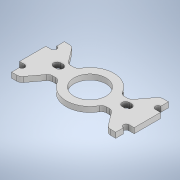
# Autodesk Inventor part: Ankle_middle_frame
Saved by Autodesk Inventor 2020.4 (Build 244396000, 396)
## iProperties
Created: 2021-10-01
Part Number: Ankle_middle_frame
Material: アルミニウム 2014-T4
Document SubType Name: Modeling
Designer: Masato Kubotera
Density: 2.8 g/cm^3
Appearance: 滑らか - 淡い灰色
Description: A2017 T2
Author: Masato Kubotera
Autodesk Inventor part; units mm, degrees
ref_plane "YZ Plane" through (0, 0, 0) normal (1, 0, 0) x (0, 1, 0)
ref_plane "XZ Plane" through (0, 0, 0) normal (0, 1, 0) x (-1, 0, 0)
ref_plane "XY Plane" through (0, 0, 0) normal (0, 0, 1) x (1, 0, 0)
sketch "スケッチ1" plane through (0, 0, 0) normal (0, 0, 1) x (1, 0, 0)
  line L0 (-19.75, 10) -> (19.75, 10) construction
  line L1 (19.75, 10) -> (19.75, -10) construction
  line L2 (19.75, -10) -> (-19.75, -10) construction
  line L3 (-19.75, -10) -> (-19.75, 10) construction
  line L4 (-19.75, 10) -> (19.75, -10) construction
  line L5 (19.75, 10) -> (-19.75, -10) construction
  line L6 (-19.75, 5) -> (-21.75, 5)
  line L7 (-21.75, 5) -> (-21.75, -5)
  line L8 (-19.75, 0) -> (19.75, 0) construction
  line L9 (0, 10) -> (0, -10) construction
  arc A0 (-19.75, 5) -> (-19.75, 7.1) centre (-19.75, 6.05) ccw
  line L10 (-16.75, 10) -> (-11.75, 3.4)
  line L11 (-19.75, -5) -> (-21.75, -5)
  arc A1 (-19.75, -7.1) -> (-19.75, -5) centre (-19.75, -6.05) ccw
  line L12 (-16.75, -10) -> (-11.75, -3.4)
  line L13 (-19.75, 7.1) -> (-19.75, 10)
  line L14 (-16.75, 10) -> (-19.75, 10)
  line L15 (-16.75, -10) -> (-19.75, -10)
  line L16 (-19.75, -7.1) -> (-19.75, -10)
  line L17 (19.75, 5) -> (21.75, 5)
  line L18 (21.75, 5) -> (21.75, -5)
  arc A2 (19.75, 7.1) -> (19.75, 5) centre (19.75, 6.05) ccw
  line L19 (16.75, 10) -> (11.75, 3.4)
  line L20 (19.75, -5) -> (21.75, -5)
  arc A3 (19.75, -5) -> (19.75, -7.1) centre (19.75, -6.05) ccw
  line L21 (16.75, -10) -> (11.75, -3.4)
  line L22 (19.75, 7.1) -> (19.75, 10)
  line L23 (16.75, 10) -> (19.75, 10)
  line L24 (16.75, -10) -> (19.75, -10)
  line L25 (19.75, -7.1) -> (19.75, -10)
  arc A4 (8.387, 3.4) -> (-8.387, 3.4) centre (0, 0) ccw
  arc A5 (-8.387, -3.4) -> (8.387, -3.4) centre (0, 0) ccw
  line L26 (-11.75, 3.4) -> (-8.387, 3.4)
  line L27 (-8.387, -3.4) -> (-11.75, -3.4)
  line L28 (8.387, -3.4) -> (11.75, -3.4)
  line L29 (11.75, 3.4) -> (8.387, 3.4)
  circle A6 centre (0, 0) radius 6 construction
  circle A7 centre (0, 0) radius 6.05
  arc A8 (-13.5, 2.35) -> (-13.5, -0.35) centre (-13.5, 1) ccw
  line L30 (-13.5, 1) -> (13.5, 1) construction
  line L31 (-13.5, 2.35) -> (-12.5, 2.35)
  line L32 (-12.5, -0.35) -> (-13.5, -0.35)
  arc A9 (-12.5, -0.35) -> (-12.5, 2.35) centre (-12.5, 1) ccw
  circle A10 centre (-13.5, 1) radius 2.4 construction
  arc A11 (13.5, -0.35) -> (13.5, 2.35) centre (13.5, 1) ccw
  arc A12 (12.5, 2.35) -> (12.5, -0.35) centre (12.5, 1) ccw
  line L33 (12.5, 2.35) -> (13.5, 2.35)
  line L34 (12.5, -0.35) -> (13.5, -0.35)
  point P0 (0, 0)
  point P1 (0, 1)
  dimension "d0" = 39.5
  dimension "d4" = 2
  dimension "d5" = 10
  dimension "d6" = 1.05
  dimension "d7" = 3
  dimension "d9" = 5
  dimension "d11" = 8
  dimension "d26" = 12
  dimension "d27" = 0.05
  dimension "d28" = 12.1
  dimension "d30" = 27
  dimension "d32" = 1
  dimension "d33" = 1.35
  dimension "d34" = 1
  dimension "d35" = 4.8
  dimension "d36" = 3
  constraints: 70 end point, 26 symmetric about line, 20 point on circle, 13 centre point, 11 midpoint, 6 parallel, 6 point on line, 5 horizontal, 5 tangent, 3 coincident, 3 perpendicular, 2 collinear, 6 other
  measures "d0" distance of L1.end L2.end
  measures "d4" distance of L6.start L6.end
  measures "d5" distance of L6.end L7.end
  measures "d6" radius of A0
  measures "d7" distance of L10.start L0.start
  measures "d9" vertical distance of L6.end L0.start
  measures "d11" horizontal distance of L0.start L10.end
  measures "d26" diameter of A6
  measures "d27" radial gap between concentric circles of A7 A6
  measures "d28" diameter of A7
  measures "d30" distance of L30.start L30.end
  measures "d32" distance of L30.start A9.centre
  measures "d33" radius of A8
  measures "d34" distance of point (0, 0) point (0, 1)
  measures "d35" diameter of A10
  measures "d36" radial gap between concentric circles of A4 A7
extrude "押し出し1" add sketch "スケッチ1" along normal blind 2
fillet "フィレット1" radius 2 12 edges at (-11.75, 3.4, 1) (-11.75, -3.4, 1) (-16.75, 10, 1) (-16.75, -10, 1) (-8.387, -3.4, 1) (-8.387, 3.4, 1) (8.387, 3.4, 1) (8.387, -3.4, 1) (11.75, 3.4, 1) (11.75, -3.4, 1) (16.75, 10, 1) (16.75, -10, 1)
